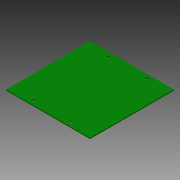
# Autodesk Inventor part: CompCellScopeArray
Saved by Autodesk Inventor 2015 (Build 190159000, 159)
## iProperties
Created: 2015-03-24
Part Number: CompCellScopeArray
Material: Generic
Document SubType Name: Modeling
Designer: Nitin
Density: 1 g/cm^3
Appearance: Default
Author: Nitin
Autodesk Inventor part; units mm, degrees
ref_plane "YZ Plane" through (0, 0, 0) normal (1, 0, 0) x (0, 1, 0)
ref_plane "XZ Plane" through (0, 0, 0) normal (0, 1, 0) x (-1, 0, 0)
ref_plane "XY Plane" through (0, 0, 0) normal (0, 0, 1) x (1, 0, 0)
sketch "Sketch3" plane through (0, 0, 0) normal (0, 1, 0) x (-1, 0, 0)
  line L0 (50, 50) -> (-50, 50)
  line L1 (-50, 50) -> (-50, -50)
  line L2 (-50, -50) -> (50, -50)
  line L3 (50, -50) -> (50, 50)
  line L4 (-50, -45) -> (50, -45) construction
  line L5 (-50, 45) -> (50, 45) construction
  line L6 (22.5, 50) -> (22.5, -50) construction
  line L7 (-22.5, 50) -> (-22.5, -50) construction
  circle A0 centre (-22.5, -45) radius 1.575
  circle A1 centre (-22.5, 45) radius 1.575
  circle A2 centre (22.5, 45) radius 1.575
  circle A3 centre (22.5, -45) radius 1.575
  point P0 (0, 0)
  dimension "d4" = 100
  dimension "d5" = 100
  dimension "d6" = 5
  dimension "d7" = 5
  dimension "d8" = 27.5
  dimension "d9" = 27.5
  dimension "d10" = 3.15
  dimension "d11" = 3.15
  dimension "d12" = 3.15
  dimension "d13" = 3.15
  constraints: 16 end point, 16 point on line, 4 centre point, 3 parallel, 3 perpendicular, 1 horizontal, 1 vertical
  measures "d4" distance of L1.end L2.end
  measures "d5" distance of L2.end L0.start
  measures "d6" distance between parallel lines of L2 L4
  measures "d7" distance between parallel lines of L0 L5
  measures "d8" distance between parallel lines of L6 L3
  measures "d9" distance between parallel lines of L1 L7
  measures "d10" diameter of A0
  measures "d11" diameter of A1
  measures "d12" diameter of A2
  measures "d13" diameter of A3
extrude "Extrusion1" add sketch "Sketch3" along normal blind 1
body "Solid1"
